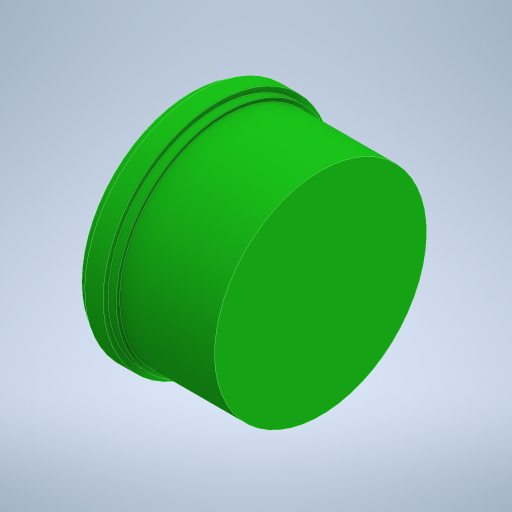
# Autodesk Inventor part: prop_meter
Saved by Autodesk Inventor 2024.2 (Build 282272000, 272)
## iProperties
Created: 2025-03-01
Part Number: prop_meter
Material: Všeobecné
Document SubType Name: Modeling
Designer: hepma_axt67em
Density: 1 g/cm^3
Appearance: Tmavě zelená
Author: hepma_axt67em
Autodesk Inventor part; units mm, degrees
ref_plane "YZ Plane" through (0, 0, 0) normal (1, 0, 0) x (0, 1, 0)
ref_plane "XZ Plane" through (0, 0, 0) normal (0, 1, 0) x (-1, 0, 0)
ref_plane "XY Plane" through (0, 0, 0) normal (0, 0, 1) x (1, 0, 0)
sketch "Náčrt1" plane through (0, 0, 0) normal (0, 0, 1) x (1, 0, 0)
  line L0 (-42.48, 0) -> (7.08, 0) projected
  line L1 (0, 37.68) -> (0, -6.28) projected
  line L2 (-35.4, 0) -> (0, 0)
  line L3 (-35.4, 0) -> (-35.4, 30)
  line L4 (-35.4, 30) -> (-33.2, 30)
  line L5 (-33.2, 30) -> (-33.2, 31.4)
  line L6 (-33.2, 31.4) -> (-28.2, 31.4)
  line L7 (-28.2, 31.4) -> (-28.2, 30)
  line L8 (-28.2, 30) -> (-26, 30)
  line L9 (-26, 30) -> (-26, 29.05)
  line L10 (-26, 29.05) -> (0, 29.05)
  line L11 (0, 29.05) -> (0, 0)
  point P0 (0, 0)
  point P1 (0, 29.05)
  dimension "d1" = 29.05
  dimension "d2" = 30
  dimension "d3" = 31.4
  dimension "d4" = 35.4
  dimension "d5" = 2.2
  dimension "d6" = 2.2
  dimension "d7" = 5
  constraints: 20 end point, 7 perpendicular, 2 collinear, 2 point on line, 1 horizontal, 1 vertical
  measures "d1" distance of L10.end L2.end
  measures "d2" distance between parallel lines of L2 L8
  measures "d3" distance between parallel lines of L2 L6
  measures "d4" distance of L2.start L2.end
  measures "d5" distance of L7.end L8.end
  measures "d6" distance of L3.end L4.end
  measures "d7" distance of L5.end L6.end
revolve "Rotace1" add sketch "Náčrt1" angle 360 about axis through (0, 0, 0) along (1, 0, 0)
